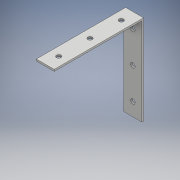
# Autodesk Inventor part: 100mmX20mmCornerBracket
Saved by Autodesk Inventor 2017 (Build 210142000, 142)
## iProperties
Created: 2017-10-02
Part Number: 100mmX20mmCornerBracket
Material: Generic
Document SubType Name: Modeling
Designer: Kathryn Rosie
Density: 1 g/cm^3
Appearance: Default
Author: Kathryn Rosie
Autodesk Inventor part; units mm, degrees
ref_plane "YZ Plane" through (0, 0, 0) normal (1, 0, 0) x (0, 1, 0)
ref_plane "XZ Plane" through (0, 0, 0) normal (0, 1, 0) x (-1, 0, 0)
ref_plane "XY Plane" through (0, 0, 0) normal (0, 0, 1) x (1, 0, 0)
sketch "Sketch1" plane through (0, 0, 0) normal (1, 0, 0) x (0, 1, 0)
  line L0 (0, -0.2) -> (0, -100)
  line L1 (0, -100) -> (-2, -100)
  line L2 (-2, -100) -> (-2, -2.2)
  line L3 (-2.2, -2) -> (-100, -2)
  line L4 (-100, -2) -> (-100, 0)
  line L5 (-100, 0) -> (-0.2, 0)
  arc A0 (-2, -2.2) -> (-2.2, -2) centre (-2.2, -2.2) ccw
  arc A1 (0, -0.2) -> (-0.2, 0) centre (-0.2, -0.2) ccw
  point P0 (0, 0)
  point P1 (-2, -2)
  dimension "d0" = 100
  dimension "d1" = 2
  dimension "d2" = 98
  dimension "d3" = 98
  dimension "d4" = 2
  dimension "d5" = 0.2
  constraints: 12 end point, 4 perpendicular, 4 point on circle, 4 point on line, 4 tangent, 2 centre point, 1 equal radius, 1 vertical
  measures "d0" distance of point (0, 0) L0.end
  measures "d1" distance of L0.end L1.end
  measures "d2" distance of L1.end point (-2, -2)
  measures "d3" distance of point (-2, -2) L3.end
  measures "d4" distance of L3.end L4.end
  measures "d5" radius of A0
extrude "Extrusion1" add sketch "Sketch1" along normal blind 20
sketch "Sketch2" plane through (0, 0, -0.2) normal (0, 1, 0) x (1, 0, 0)
  line L0 (0, 99.8) -> (20, 99.8) projected
  line L1 (10, 99.8) -> (10, 2)
  line L2 (0, 2) -> (20, 2) projected
  line L3 (0, -0.2) -> (20, -0.2) projected
  point P0 (10, 14.8)
  point P1 (10, 49.8)
  point P2 (10, 84.8)
  dimension "d9" = 15
  dimension "d10" = 35
  dimension "d11" = 35
  constraints: 3 point on line, 2 end point, 2 midpoint
  measures "d9" distance from line of L3 point (10, 14.8)
  measures "d10" distance of point (10, 49.8) point (10, 14.8)
  measures "d11" distance of point (10, 84.8) point (10, 49.8)
hole "Hole1" at (10, 0, -15) at (10, 0, -50) at (10, 0, -85) direction (0, -1, 0) diameter 5 end through all
sketch "Sketch3" plane through (0, -100, 0) normal (0, 0, 1) x (1, 0, 0)
  line L0 (0, 0) -> (20, 0) projected
  line L1 (10, 0) -> (10, 99.8)
  line L2 (0, 99.8) -> (20, 99.8) projected
  point P0 (0, 100)
  point P1 (10, 15)
  point P2 (10, 50)
  point P3 (10, 85)
  dimension "d19" = 15
  dimension "d20" = 35
  dimension "d21" = 35
  constraints: 3 point on line, 2 end point, 2 midpoint
  measures "d19" distance of point (10, 15) L1.start
  measures "d20" distance of point (10, 50) point (10, 15)
  measures "d21" distance of point (10, 85) point (10, 50)
hole "Hole2" at (10, -85, 0) at (10, -50, 0) at (10, -15, 0) direction (0, 0, -1) diameter 5 end through all
body "Solid1"
